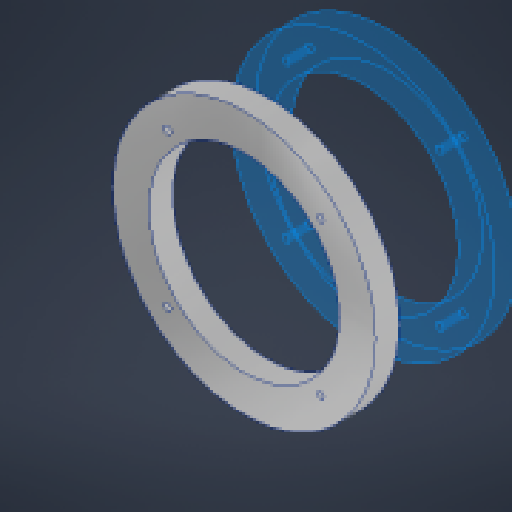
# Autodesk Inventor part: drehkranz
Saved by Autodesk Inventor 2023 (Build 270158000, 158)
## iProperties
Created: 2026-03-19
Part Number: drehkranz
Material: Aluminium 6061
Document SubType Name: Modeling
Designer: lerat
Mass: 719.664 g
Surface Area: 503.692 cm^2
Volume: 266.542 cm^3
Density: 2.7 g/cm^3
Appearance: Aluminium - flach
Author: lerat
Autodesk Inventor part; units mm, degrees
ref_plane "YZ Plane" through (0, 0, 0) normal (1, 0, 0) x (0, 1, 0)
ref_plane "XZ Plane" through (0, 0, 0) normal (0, 1, 0) x (-1, 0, 0)
ref_plane "XY Plane" through (0, 0, 0) normal (0, 0, 1) x (1, 0, 0)
sketch "Skizze1" plane through (0, 0, 0) normal (0, 0, 1) x (1, 0, 0)
  circle A0 centre (0, 0) radius 100
  circle A1 centre (0, 0) radius 72.5
  circle A2 centre (0, 0) radius 82.5 construction
  line L0 (0, 0) -> (-58.3363, 58.3363) construction
  line L1 (0, 0) -> (0, 82.5)
  circle A3 centre (-58.3363, 58.3363) radius 2.75
  circle A4 centre (-58.3363, -58.3363) radius 2.75
  circle A5 centre (58.3363, -58.3363) radius 2.75
  circle A6 centre (58.3363, 58.3363) radius 2.75
  dimension "d0" = 200
  dimension "d1" = 145
  dimension "d3" = 45
  dimension "d4" = 5.5
  dimension "d5" = 165
  dimension "d8" = 360
  constraints: 7 centre point, 4 end point, 3 coincident, 2 point on circle, 1 vertical, 9 other
  measures "d0" diameter of A0
  measures "d1" diameter of A1
  measures "d3" angle of L1 L0
  measures "d4" diameter of A3
  measures "d5" diameter of A2
extrude "Extrusion1" add sketch "Skizze1" along normal blind 18
